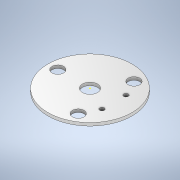
# Autodesk Inventor part: buffer
Saved by Autodesk Inventor 2020 (Build 240168000, 168)
## iProperties
Created: 2019-06-21
Part Number: buffer
Material: PBT Plastic
Document SubType Name: Modeling
Designer: ColinP
Density: 8 g/cm^3
Appearance: Clear - Light
Mass: 8.49189 g
Surface Area: 19.6339 cm^2
Volume: 1.06149 cm^3
Author: ColinP
Autodesk Inventor part; units mm, degrees
ref_plane "YZ Plane" through (0, 0, 0) normal (1, 0, 0) x (0, 1, 0)
ref_plane "XZ Plane" through (0, 0, 0) normal (0, 1, 0) x (-1, 0, 0)
ref_plane "XY Plane" through (0, 0, 0) normal (0, 0, 1) x (1, 0, 0)
sketch "Sketch1" plane through (0, 0, 0) normal (0, 1, 0) x (-1, 0, 0)
  circle A0 centre (0, 0) radius 17.78
  dimension "d0" = 35.56
  constraints: 1 centre point, 1 coincident
  measures "d0" diameter of A0
extrude "Extrusion1" add sketch "Sketch1" along normal blind 1.27
sketch "Sketch2" plane through (0, 1.27, 0) normal (0, 1, 0) x (1, 0, 0)
  circle A0 centre (0, 0) radius 17.78 projected
  constraints: 1 coincident
hole "Hole1" at (0, 1.27, 0) direction (0, -1, 0) diameter 6.35 end through all
sketch "Sketch3" plane through (0, 1.27, 0) normal (0, 1, 0) x (1, 0, 0)
  line L0 (0, 0) -> (-13.6144, 0)
  dimension "d10" = 13.6144
  constraints: 2 end point, 1 horizontal
  measures "d10" distance of L0.start L0.end
hole "Hole2" at (-13.6144, 1.27, 0) direction (0, -1, 0) diameter 4.9022 end through all
pattern_circular "Circular Pattern1" count 3 over 360 about axis through (0, -49.0355, 0) along (0, 1, 0) of "Hole2"
sketch "Sketch8" plane through (0, 1.27, 0) normal (0, 1, 0) x (1, 0, 0)
  point P0 (0, 0)
sketch "Sketch9" plane through (0, 1.27, 0) normal (0, 1, 0) x (1, 0, 0)
  line L0 (0, 0) -> (10.16, 0)
  line L1 (10.16, 0) -> (10.16, 5.08)
  line L2 (10.16, 5.08) -> (10.16, -5.08)
  dimension "d61" = 10.16
  dimension "d62" = 5.08
  dimension "d63" = 10.16
  constraints: 6 end point, 1 horizontal, 1 perpendicular, 1 point on line
  measures "d61" distance of L0.start L0.end
  measures "d62" distance of L0.end L1.end
  measures "d63" distance of L1.end L2.end
hole "Hole7" at (10.16, 1.27, -5.08) at (10.16, 1.27, 5.08) direction (0, -1, 0) diameter 1.905 end through all
sketch "Sketch10" plane through (0, 1.27, 0) normal (0, 1, 0) x (1, 0, 0)
  circle A0 centre (-13.6144, 0) radius 2.4511 projected
  line L0 (0, 0) -> (-13.6144, 0)
  line L1 (-13.6144, 0) -> (-3.175, 0)
  circle A1 centre (0, 0) radius 3.175 projected
  line L2 (0, 0) -> (-3.175, 9.6512)
  line L3 (-3.175, 9.6512) -> (0, 0)
  line L4 (0, 0) -> (-3.175, -9.6512)
  dimension "d71" = 10.16
  dimension "d72" = 10.16
  constraints: 10 end point, 1 collinear, 1 horizontal, 1 horizontal alignment, 1 point on line, 1 other
  measures "d71" distance of L2.start L2.end
  measures "d72" distance of L2.start L4.end
hole "Hole8" [suppressed]
body "Solid1"
